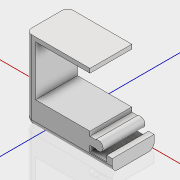
# Autodesk Inventor part: ЛЦМК.30000.10.00.02 Крышка задняя
Saved by Autodesk Inventor 2021.2 (Build 252289000, 289)
## iProperties
Created: 2025-11-22
Part Number: ЛЦМК.30000.10.00.02 Крышка задняя
Material: Типовые
Document SubType Name: Modeling
Designer: Захаров
Density: 1 g/cm^3
Appearance: По умолчанию
Author: Захаров
Autodesk Inventor part; units mm, degrees
ref_plane "YZ Plane" through (0, 0, 0) normal (1, 0, 0) x (0, 1, 0)
ref_plane "XZ Plane" through (0, 0, 0) normal (0, 1, 0) x (-1, 0, 0)
ref_plane "XY Plane" through (0, 0, 0) normal (0, 0, 1) x (1, 0, 0)
sketch "Эскиз1" plane through (0, 0, 0) normal (0, 0, 1) x (1, 0, 0)
  arc A0 (19.25, -13.5) -> (19.25, -10.5) centre (20.245, -12) ccw projected
  line L0 (19.25, -10.5) -> (17.25, -10.5) projected
  line L1 (17.25, -13.5) -> (19.25, -13.5) projected
  line L2 (17.25, -10.6) -> (19.2806, -10.6)
  arc A1 (19.2806, -13.4) -> (19.2806, -10.6) centre (20.245, -12) ccw
  line L3 (19.2806, -13.4) -> (17.25, -13.4)
  line L4 (17.25, -13.5) -> (17.25, -15.5) projected
  line L5 (17.25, 3) -> (17.25, -10.5) projected
  line L6 (19.25, -9) -> (-2.25, -9) projected
  line L7 (-2.25, -9) -> (-2.25, 9) projected
  line L8 (-2.25, 9) -> (19.25, 9) projected
  line L9 (17.25, 10.5) -> (17.25, 6.5) projected
  line L10 (17.25, 10.5) -> (-5.75, 10.5)
  line L11 (-5.75, 10.5) -> (-5.75, -17.9303)
  line L12 (23.25, -17.9303) -> (-3.75, -17.9303) projected
  line L13 (-5.75, -15.9303) -> (-5.75, 10.5) projected
  line L14 (-5.75, -17.9303) -> (-3.75, -17.9303)
  line L15 (25.25, -13.5) -> (25.25, -15.9303) projected
  line L16 (23.25, -13.5) -> (25.25, -13.5) projected
  line L17 (23.25, -15.5) -> (23.25, -13.5) projected
  line L18 (23.25, -17.9303) -> (-3.75, -17.9303) projected
  line L19 (25.25, -15.9303) -> (25.25, -17.9303)
  line L20 (25.25, -17.9303) -> (23.25, -17.9303)
  line L21 (17.25, -15.5) -> (23.25, -15.5)
  line L22 (17.25, -13.4) -> (17.25, -13.5)
  line L23 (17.25, -10.6) -> (17.25, -10.5)
  point P0 (0, 0)
  point P1 (17.25, -9)
  point P2 (17.25, 9)
  dimension "d0" = 0.1
  dimension "d1" = 23
  constraints: 20 end point, 3 horizontal, 3 perpendicular, 2 point on circle, 2 vertical, 1 centre point, 1 point on line, 2 other
  measures "d0" radial gap between concentric circles of A0 A1
  measures "d1" distance of L9.start L10.end
extrude "Выдавливание1" add sketch "Эскиз1" along normal blind 15 contours L4 L21 L17 L16 L15 L19 L20 L12 L14 L11 L10 L9 L8 L7 L6 L5 L23 L2 A1 L3 L22
fillet "Сопряжение1" radius 2 6 edges at (-5.75, -17.9303, 7.5) (-5.75, -3.7151, 0) (-5.75, -3.7151, 15) (9.75, -17.9303, 0) (9.75, -17.9303, 15) (25.25, -17.9303, 7.5)
